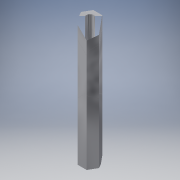
# Autodesk Inventor part: 3 in churro
Saved by Autodesk Inventor 2016 (Build 200138000, 138)
## iProperties
Created: 2016-01-16
Part Number: 3 in churro
Material: Aluminum 6061
Document SubType Name: Modeling
Designer: gus
Density: 2.7 g/cm^3
Appearance: Aluminum - Flat
Mass: 30.1377 g
Surface Area: 65.1762 cm^2
Volume: 11.1621 cm^3
User Status: complete
Author: gus
Autodesk Inventor part; units mm, degrees
ref_plane "YZ Plane" through (0, 0, 0) normal (1, 0, 0) x (0, 1, 0)
ref_plane "XZ Plane" through (0, 0, 0) normal (0, 1, 0) x (-1, 0, 0)
ref_plane "XY Plane" through (0, 0, 0) normal (0, 0, 1) x (1, 0, 0)
sketch "Sketch1" plane through (0, 0, 0) normal (0, 1, 0) x (-1, 0, 0)
  circle A0 centre (0, 0) radius 2.9337
  line L0 (-3.6295, -6.2865) -> (-7.259, 0)
  line L1 (-7.259, 0) -> (-3.6295, 6.2865)
  line L2 (-3.6295, 6.2865) -> (3.6295, 6.2865)
  line L3 (3.6295, 6.2865) -> (7.259, 0)
  line L4 (7.259, 0) -> (3.6295, -6.2865)
  line L5 (3.6295, -6.2865) -> (-3.6295, -6.2865)
  dimension "d0" = 5.8674
  dimension "d1" = 6.2865
  constraints: 12 end point, 2 coincident, 1 centre point, 1 horizontal, 13 other
  measures "d0" diameter of A0
  measures "d1" distance from line of L5 point (0, 0)
extrude "Extrusion1" add sketch "Sketch1" along normal blind 101.6
body "Solid1"
